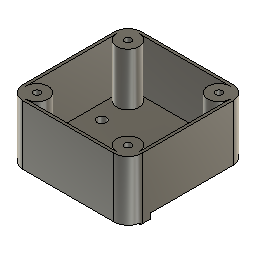
E Stop Mount (Autodesk Fusion 360 design; units mm, degrees)
Autodesk Fusion 360 part; units mm, degrees
sketch "Top" plane through (0, 0, 0) normal (0, 0, 1) x (1, 0, 0)
  line L0 (26, -26) -> (-26, -26) construction
  line L1 (-26, -26) -> (-26, 26) construction
  line L2 (-26, 26) -> (26, 26) construction
  line L3 (26, 26) -> (26, -26) construction
  line L4 (26, -26) -> (-26, 26) construction
  line L5 (-26, -26) -> (26, 26) construction
  line L6 (26, -34) -> (-26, -34)
  line L7 (-34, -26) -> (-34, 26)
  line L8 (-26, 34) -> (26, 34)
  line L9 (34, 26) -> (34, -26)
  line L10 (34, -34) -> (-34, 34) construction
  line L11 (-34, -34) -> (34, 34) construction
  arc A0 (26, -34) -> (34, -26) centre (26, -26) ccw
  arc A1 (-34, -26) -> (-26, -34) centre (-26, -26) ccw
  arc A2 (-26, 34) -> (-34, 26) centre (-26, 26) ccw
  arc A3 (34, 26) -> (26, 34) centre (26, 26) ccw
  arc A4 (26, -32.4) -> (32.4, -26) centre (26, -26) ccw
  line L12 (32.4, 26) -> (32.4, -26)
  arc A5 (32.4, 26) -> (26, 32.4) centre (26, 26) ccw
  line L13 (-26, 32.4) -> (26, 32.4)
  arc A6 (-26, 32.4) -> (-32.4, 26) centre (-26, 26) ccw
  line L14 (-32.4, -26) -> (-32.4, 26)
  arc A7 (-32.4, -26) -> (-26, -32.4) centre (-26, -26) ccw
  line L15 (26, -32.4) -> (-26, -32.4)
  circle A8 centre (-24, 9) radius 2.6
  circle A9 centre (9, -24) radius 2.6
  circle A10 centre (26, -26) radius 6.4
  circle A11 centre (26, 26) radius 6.4
  circle A12 centre (-26, 26) radius 6.4
  circle A13 centre (-26, -26) radius 6.4
  line L16 (-34, -12) -> (-12, -12) construction
  line L17 (-12, -12) -> (-12, -34) construction
  circle A14 centre (-12, -12) radius 2.5
  circle A15 centre (-24, 9) radius 5
  circle A16 centre (9, -24) radius 5
  line L18 (34, -21) -> (-21, -21)
  line L19 (-21, -21) -> (-21, 34)
  line L20 (34, -27) -> (-27, -27)
  line L21 (-27, -27) -> (-27, 34)
  line L22 (-13.5, -34) -> (-13.5, -13.5)
  line L23 (-13.5, -13.5) -> (-34, -13.5)
  circle A17 centre (-24, -24) radius 2
  point P0 (26, -26)
  dimension "d1" = 52
  dimension "d2" = 52
  dimension "d3" = 68
  dimension "d4" = 68
  dimension "d5" = 8
  dimension "d6" = 8
  dimension "d7" = 8
  dimension "d8" = 8
  dimension "d9" = 1.6
  dimension "d14" = 5.2
  dimension "d15" = 10
  dimension "d16" = 5.2
  dimension "d17" = 10
  dimension "d18" = 22
  dimension "d19" = 22
  dimension "d20" = 5
  dimension "d25" = 10
  dimension "d26" = 10
  dimension "d34" = 13
  dimension "d35" = 13
  dimension "d36" = 6
  dimension "d43" = 20.5
  dimension "d44" = 20.5
  dimension "d48" = 25
  dimension "d49" = 25
  dimension "d50" = 4
  dimension "d51" = 10
  dimension "d52" = 10
  constraint perpendicular L0 L1
  constraint parallel L0 L2
  constraint parallel L1 L3
  constraint horizontal L0
  constraint coincident L4 origin
  constraint coincident L5 origin
  constraint perpendicular L6 L7
  constraint parallel L6 L8
  constraint parallel L7 L9
  constraint horizontal L6
  constraint coincident L10 origin
  constraint coincident L11 origin
  constraint tangent L9 A0
  constraint tangent L6 A0
  constraint coincident L11.start L6
  constraint coincident L11.start L7
  constraint tangent L6 A1
  constraint tangent L7 A1
  constraint coincident L10.end L8
  constraint coincident L10.end L7
  constraint tangent L8 A2
  constraint tangent L7 A2
  constraint coincident L11.end L9
  constraint coincident L11.end L8
  constraint tangent L9 A3
  constraint tangent L8 A3
  constraint coincident P0 L0.start
  constraint coincident L2.end L3.start
  constraint concentric A2 A12
  constraint coincident L0.end L1.start
  constraint coincident L7 L16.start
  constraint coincident L6 L17.end
  constraint perpendicular L6 L17
  constraint coincident L16.end L17.start
  constraint perpendicular L7 L16
  constraint concentric A8 A15
  constraint concentric A9 A16
  constraint coincident L9 L18.start
  constraint perpendicular L17 L18
  constraint coincident L8 L19.end
  constraint perpendicular L8 L19
  constraint coincident L6 L22.start
  constraint perpendicular L18 L22
  constraint coincident L7 L23.end
  constraint perpendicular L7 L23
  measures "d1" distance of L1.end L2.end
  measures "d2" distance of L0.end L1.end
  measures "d3" distance of L10.end L11.end
  measures "d4" distance of L11.start L10.end
  measures "d5" radius of A0
  measures "d6" radius of A1
  measures "d7" radius of A2
  measures "d8" radius of A3
  measures "d14" diameter of A8
  measures "d15" distance of L7 A8.centre
  measures "d16" diameter of A9
  measures "d17" distance of L6 A9.centre
  measures "d18" distance of L16.start L16.end
  measures "d19" distance of L16.end L17.end
  measures "d20" diameter of A14
  measures "d25" diameter of A15
  measures "d26" diameter of A16
  measures "d34" distance of L7 L19
  measures "d35" distance of L6 L18
  measures "d43" distance of L6 L23
  measures "d44" distance of L7 L22
  measures "d48" distance of L9 A9.centre
  measures "d49" distance of L8 A8.centre
  measures "d50" diameter of A17
  measures "d51" distance of L6 A17.centre
  measures "d52" distance of L7 A17.centre
extrude "Extrude1" add sketch "Top" along normal blind 2 contours L6 A0 A4 L15 A10 L20 L22 | L6 L7 A1 L14 A7 L15 A13 L22 L23 | L9 A0 A4 L12 A10 L18 L20 | L15 A10 A16 L20 L22 | L15 A13 L20 L22 | A4 A10 L18 L20 | A4 A10 L20 | A7 A13 L20 L21 | A16 L18 L20 L22 | A13 L18 L19 L20 L21 L22 L23 | L8 L9 A3 L12 A5 L13 A11 L18 L19 | L12 A10 L18 | A10 A16 L18 L20 | L7 A2 A6 L14 A12 L21 L23 | L14 A13 L21 L23 | A13 L20 L21 | A16 L20 | A16 L18 L20 | L12 L13 A10 A11 A12 A14 A15 A16 L18 L19 L22 L23 | A14 L18 L19 L22 L23 | A10 L18 | L14 A12 A15 L21 L23 | A16 L18 | L8 A2 L13 A6 A12 L19 L21 | A6 A12 L21 | A15 L19 L21 L23 | A6 A12 L19 L21 | A12 A15 L19 L21 | A15 L19 L21 | A15 L21 | A15 L19 | L13 A12 L19 | A12 L19 | A17
extrude "Extrude2" add sketch "Top" along normal blind 32 contours L6 A0 A4 L15 A10 L20 L22 | L6 L7 A1 L14 A7 L15 A13 L22 L23 | L9 A0 A4 L12 A10 L18 L20 | A4 A10 L18 L20 | A4 A10 L20 | A7 A13 L20 L21 | L8 L9 A3 L12 A5 L13 A11 L18 L19 | L7 A2 A6 L14 A12 L21 L23 | A13 L20 L21 | A10 L18 | A5 A11 | L8 A2 L13 A6 A12 L19 L21 | A6 A12 L21 | A6 A12 L19 L21 | A12 L19 | A17
extrude "Extrude3" add sketch "Top" along normal blind 2 contours A16 L20 | A16 L18 L20 | A16 L18 | A15 L19 L21 | A15 L21 | A15 L19
extrude "Extrude5" add sketch "Top" against normal blind 2 contours L6 A0 A4 L15 A10 L20 L22 | L6 L7 A1 L14 A7 L15 A13 L22 L23 | L15 A10 A16 L20 L22 | L15 A13 L20 L22 | A4 A10 L20 | A7 A13 L20 L21 | A13 L18 L19 L20 L21 L22 L23 | L7 A2 A6 L14 A12 L21 L23 | L14 A13 L21 L23 | A13 L20 L21 | A16 L20 | L14 A12 A15 L21 L23 | A6 A12 L21 | A15 L21 | A17
extrude "Extrude6" add sketch "Top" against normal blind 3 contours L9 A0 A4 L12 A10 L18 L20 | A4 A10 L18 L20 | A16 L18 L20 L22 | L12 A10 L18 | A10 A16 L18 L20 | A16 L18 L20 | L8 A2 L13 A6 A12 L19 L21 | A15 L19 L21 L23 | A6 A12 L19 L21 | A12 A15 L19 L21 | A15 L19 L21 | L13 A12 L19
sketch "Sketch3" plane through (0, 0, 32) normal (0, 0, 1) x (-1, 0, 0)
  line L0 (-26, 32.4) -> (26, 32.4)
  arc A0 (26, 32.4) -> (32.4, 26) centre (26, 26) ccw
  line L1 (32.4, 26) -> (32.4, -26)
  arc A1 (32.4, -26) -> (26, -32.4) centre (26, -26) ccw
  line L2 (26, -32.4) -> (-26, -32.4)
  arc A2 (-26, -32.4) -> (-32.4, -26) centre (-26, -26) ccw
  line L3 (-32.4, -26) -> (-32.4, 26)
  arc A3 (-32.4, 26) -> (-26, 32.4) centre (-26, 26) ccw
  arc A4 (-26, 34) -> (-34, 26) centre (-26, 26) ccw
  line L4 (-34, 26) -> (-34, -26)
  arc A5 (-34, -26) -> (-26, -34) centre (-26, -26) ccw
  line L5 (-26, -34) -> (26, -34)
  arc A6 (26, -34) -> (34, -26) centre (26, -26) ccw
  line L6 (34, -26) -> (34, 26)
  arc A7 (34, 26) -> (26, 34) centre (26, 26) ccw
  line L7 (26, 34) -> (-26, 34)
  point P0 (26, 26)
  point P1 (-26, 26)
  point P2 (-26, -26)
  point P3 (26, -26)
  constraint coincident P0 A0.centre
  constraint coincident P1 A3.centre
  constraint coincident P2 A2.centre
  constraint coincident P3 A1.centre
hole "Hole1" at (-26, -26, 32) at (-26, 26, 32) at (26, 26, 32) at (26, -26, 32) direction (0, 0, -1) diameter 3.9 depth 15 tip angle 118
extrude "Extrude8" cut sketch "Top" against normal up to surface (2 mm away) contours A17
ref_plane "WorkPlane1" through (-22.0781, -20.9425, 27.0049) normal (0.612802, 0.790236, 0) x (0.790236, -0.612802, 0)
sketch "Sketch4" plane through (-22.0781, -20.9425, 27.0049) normal (0.612802, 0.790236, 0) x (0.790236, -0.612802, 0)
  circle A0 centre (0, 21.0049) radius 3
  line L0 (6.4, 25.0049) -> (-6.4, 25.0049)
  dimension "d56" = 6
  dimension "d57" = 4
  measures "d56" diameter of A0
  measures "d57" distance of A0.centre L0
loft "Loft1" cut profiles "Sketch4", "Top" section 1 section 2 contours A17
